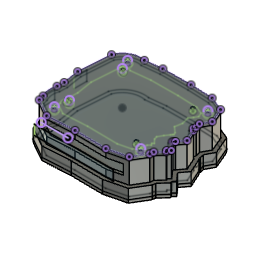
PCBPWM_v2 v1 (Autodesk Fusion 360 design; units mm, degrees)
Autodesk Fusion 360 part; units mm, degrees
sketch "pwm_pcb_larger-NPTH-drl_map" plane through (-62.4412, 140.8247, 0) normal (0, 0, 1) x (1, 0, 0)
  line L0 (167.8, -97.8) -> (171.4, -101.8)
  line L1 (171.4, -104.8) -> (169.4, -107)
  line L2 (85.4, -80) -> (87.4, -51.8)
  line L3 (122.4, -120.6) -> (98.6, -122)
  line L4 (94.9432, -49.9251) -> (114, -47.8)
  line L5 (88, -96.2) -> (85.4, -80)
  line L6 (168.6, -59) -> (166.2, -62.4)
  line L7 (173, -84.8) -> (172.2, -86)
  line L8 (141.4, -47.6) -> (161.2, -48.4)
  line L9 (172.2, -86) -> (169.4, -90)
  line L10 (169.4, -107) -> (168.8, -112)
  line L11 (170.4, -55.6) -> (168.6, -59)
  line L12 (168.8, -112) -> (165.2, -118)
  line L13 (171.4, -101.8) -> (170.2, -103)
  line L14 (166.2, -62.4) -> (168.2, -69.8)
  line L15 (172.6, -81.8) -> (173.6, -84)
  line L16 (89.2, -108.4) -> (92.4, -111.6)
  arc A0 (94.9432, -49.9251) -> (87.4, -51.8) centre (92.2153, -55.0617) ccw
  line L17 (92.4, -108.4) -> (89.2, -111.6)
  line L18 (91.491, -53.264) -> (94.691, -56.464)
  line L19 (166.8, -94.8) -> (167.8, -97.8)
  line L20 (114, -47.8) -> (141.4, -47.6)
  line L21 (161.2, -48.4) -> (168.6, -51.4)
  arc A1 (87.5716, -106.689) -> (88.2, -114.2) centre (93.4337, -109.9803) ccw
  line L22 (164.8, -110.2) -> (161.6, -113.4)
  line L23 (161.6, -110.2) -> (164.8, -113.4)
  line L24 (153, -121) -> (122.4, -120.6)
  line L25 (161.2, -52.2) -> (164.4, -55.4)
  line L26 (170.2, -103) -> (171.4, -104.8)
  line L27 (168.2, -69.8) -> (167, -76.8)
  line L28 (165.2, -118) -> (153, -121)
  line L29 (164.4, -52.2) -> (161.2, -55.4)
  line L30 (98.6, -122) -> (88.8, -116.4)
  line L31 (168.6, -51.4) -> (170.4, -55.6)
  line L32 (89.2, -108.4) -> (92.4, -111.6)
  line L33 (173.6, -84) -> (173, -84.8)
  line L34 (94.691, -53.264) -> (91.491, -56.464)
  line L35 (92.4, -108.4) -> (89.2, -111.6)
  line L36 (169.4, -90) -> (166.8, -94.8)
  line L37 (87.5716, -106.689) -> (88, -96.2)
  line L38 (167, -76.8) -> (172.6, -81.8)
  line L39 (88.8, -116.4) -> (88.2, -114.2)
  circle A2 centre (90.8, -110) radius 1.6
  circle A3 centre (163.2, -111.8) radius 1.6
  circle A4 centre (162.8, -53.8) radius 1.6
  circle A5 centre (93.091, -54.864) radius 1.6
  line L40 (176.1705, -43.6786) -> (181.4744, -56.0543)
  line L41 (181.4744, -56.0543) -> (177.1386, -64.2442)
  line L42 (177.1386, -64.2442) -> (177.0798, -64.3276)
  line L43 (177.0798, -64.3276) -> (178.4285, -69.318)
  line L44 (178.4285, -69.318) -> (177.7922, -73.0299)
  line L45 (177.7922, -73.0299) -> (180.8318, -75.7439)
  line L46 (180.8318, -75.7439) -> (185.1564, -85.2581)
  line L47 (185.1564, -85.2581) -> (181.1665, -90.5779)
  line L48 (181.1665, -90.5779) -> (180.4575, -91.6415)
  line L49 (180.4575, -91.6415) -> (178.3809, -94.6081)
  line L50 (178.3809, -94.6081) -> (185.1798, -102.1624)
  line L51 (185.1798, -102.1624) -> (183.068, -104.2742)
  line L52 (183.068, -104.2742) -> (184.0515, -105.7495)
  line L53 (184.0515, -105.7495) -> (178.9482, -111.3631)
  line L54 (178.9482, -111.3631) -> (178.4742, -115.3128)
  line L55 (178.4742, -115.3128) -> (171.6322, -126.7162)
  line L56 (171.6322, -126.7162) -> (154.147, -131.0158)
  line L57 (154.147, -131.0158) -> (122.6286, -130.6038)
  line L58 (122.6286, -130.6038) -> (96.2196, -132.1573)
  line L59 (96.2196, -132.1573) -> (80.2422, -123.0274)
  line L60 (80.2422, -123.0274) -> (78.976, -118.3845)
  arc A6 (77.6551, -104.4404) -> (78.976, -118.3845) centre (93.4337, -109.9803) ccw
  line L61 (77.6551, -104.4404) -> (77.9674, -96.7942)
  line L62 (77.9674, -96.7942) -> (75.3434, -80.4445)
  line L63 (75.3434, -80.4445) -> (77.5665, -49.0987)
  arc A7 (96.1108, -39.7329) -> (77.5665, -49.0987) centre (92.2153, -55.0617) ccw
  line L64 (96.1108, -39.7329) -> (113.4078, -37.8041)
  line L65 (113.4078, -37.8041) -> (141.5655, -37.5985)
  line L66 (141.5655, -37.5985) -> (163.3435, -38.4784)
  line L67 (163.3435, -38.4784) -> (176.1705, -43.6786)
  line L68 (180.2893, -64.7046) -> (181.4971, -69.1733)
  line L69 (181.4971, -69.1733) -> (181.0298, -71.8989)
  line L70 (181.0298, -71.8989) -> (183.3013, -73.927)
  line L71 (183.3013, -73.927) -> (188.6234, -85.6355)
  line L72 (188.6234, -85.6355) -> (183.6165, -92.3113)
  line L73 (183.6165, -92.3113) -> (182.9347, -93.334)
  line L74 (182.9347, -93.334) -> (182.2065, -94.3743)
  line L75 (182.2065, -94.3743) -> (189.3137, -102.2711)
  line L76 (189.3137, -102.2711) -> (186.9283, -104.6564)
  line L77 (186.9283, -104.6564) -> (187.8469, -106.0343)
  line L78 (187.8469, -106.0343) -> (181.8126, -112.672)
  line L79 (181.8126, -112.672) -> (181.3765, -116.3067)
  line L80 (181.3765, -116.3067) -> (173.5618, -129.3311)
  line L81 (173.5618, -129.3311) -> (154.4911, -134.0206)
  line L82 (154.4911, -134.0206) -> (122.6971, -133.605)
  line L83 (122.6971, -133.605) -> (95.5055, -135.2045)
  line L84 (95.5055, -135.2045) -> (77.6749, -125.0156)
  line L85 (77.6749, -125.0156) -> (76.1807, -119.5368)
  arc A8 (74.6751, -103.8887) -> (76.1807, -119.5368) centre (93.4337, -109.9803) ccw
  line L86 (74.6751, -103.8887) -> (74.9576, -96.9725)
  line L87 (74.9576, -96.9725) -> (72.3264, -80.5778)
  line L88 (72.3264, -80.5778) -> (74.6063, -48.4312)
  arc A9 (96.2964, -36.6936) -> (74.6063, -48.4312) centre (92.2153, -55.0617) ccw
  line L89 (96.2964, -36.6936) -> (113.2301, -34.8053)
  line L90 (113.2301, -34.8053) -> (141.6151, -34.5981)
  line L91 (141.6151, -34.5981) -> (163.9865, -35.502)
  line L92 (163.9865, -35.502) -> (178.4417, -41.3622)
  line L93 (178.4417, -41.3622) -> (184.7967, -56.1906)
  line L94 (184.7967, -56.1906) -> (180.2893, -64.7046)
  circle A10 centre (172.2599, -116.3067) radius 4.1 construction
  circle A11 centre (91.3496, -123.3578) radius 4.1 construction
  circle A12 centre (87.8304, -45.2941) radius 4.1 construction
  circle A13 centre (173.0302, -48.7764) radius 4.1 construction
  circle A14 centre (172.2599, -116.3067) radius 2
  circle A15 centre (173.0302, -48.7764) radius 2
  circle A16 centre (87.8304, -45.2941) radius 2
  circle A17 centre (91.3496, -123.3578) radius 2
  dimension "d1" = 3.2
  dimension "d2" = 3.2
  dimension "d3" = 3.2
  dimension "d4" = 3.2
  dimension "d5" = -10
  dimension "d6" = -13
  dimension "d11" = 8.2
  dimension "d12" = 8.2
  dimension "d13" = 8.2
  dimension "d14" = 8.2
  dimension "d15" = 4
  dimension "d16" = 4
  dimension "d17" = 4
  dimension "d18" = 4
  constraint midpoint L16 A2.centre
  constraint midpoint L23 A3.centre
  constraint midpoint L25 A4.centre
  constraint midpoint L18 A5.centre
  constraint concentric A10 A14
  constraint concentric A13 A15
  constraint concentric A12 A16
  constraint concentric A11 A17
  measures "d1" diameter of A2
  measures "d2" diameter of A3
  measures "d3" diameter of A5
  measures "d4" diameter of A4
  measures "d11" diameter of A10
  measures "d12" diameter of A11
  measures "d13" diameter of A12
  measures "d14" diameter of A13
  measures "d15" diameter of A14
  measures "d16" diameter of A15
  measures "d17" diameter of A16
  measures "d18" diameter of A17
extrude "Extrude1" add sketch "pwm_pcb_larger-NPTH-drl_map" against normal blind 31.75 contours L68 L69 L70 L71 L72 L73 L74 L75 L76 L77 L78 L79 L80 L81 L82 L83 L84 L85 A8 L86 L87 L88 A9 L89 L90 L91 L92 L93 L94 makes body 1
extrude "Extrude2" add sketch "pwm_pcb_larger-NPTH-drl_map" along normal blind 3 contours L0 L1 L2 L3 L4 L5 L6 L7 L8 L9 L10 L11 L12 L13 L14 L15 A0 L19 L20 L21 A1 L24 L26 L27 L28 L30 L31 L33 L36 L37 L38 L39 | L40 L41 L42 L43 L44 L45 L46 L47 L48 L49 L50 L51 L52 L53 L54 L55 L56 L57 L58 L59 L60 A6 L61 L62 L63 A7 L64 L65 L66 L67 | L68 L69 L70 L71 L72 L73 L74 L75 L76 L77 L78 L79 L80 L81 L82 L83 L84 L85 A8 L86 L87 L88 A9 L89 L90 L91 L92 L93 L94 bodies 1
sketch "Sketch2" plane through (0, 0, 3) normal (0, 0, 1) x (1, 0, 0)
  circle A0 centre (28.3588, 30.8247) radius 1.6
  circle A1 centre (100.7588, 29.0247) radius 1.6
  circle A2 centre (100.3588, 87.0247) radius 1.6
  circle A3 centre (30.6498, 85.9607) radius 1.6
  circle A4 centre (25.3892, 95.5306) radius 2
  circle A5 centre (110.589, 92.0483) radius 2
  circle A6 centre (28.9085, 17.467) radius 2
  circle A7 centre (109.8187, 24.518) radius 2
  arc A8 (33.8553, 104.1311) -> (12.1651, 92.3936) centre (29.7742, 85.763) ccw
  line L0 (12.1651, 92.3936) -> (9.8852, 60.2469)
  line L1 (9.8852, 60.2469) -> (12.5165, 43.8523)
  line L2 (12.5165, 43.8523) -> (12.234, 36.936)
  arc A9 (12.234, 36.936) -> (13.7395, 21.2879) centre (30.9925, 30.8444) ccw
  line L3 (13.7395, 21.2879) -> (15.2337, 15.8092)
  line L4 (15.2337, 15.8092) -> (33.0644, 5.6202)
  line L5 (33.0644, 5.6202) -> (60.256, 7.2197)
  line L6 (60.256, 7.2197) -> (92.05, 6.8041)
  line L7 (92.05, 6.8041) -> (111.1207, 11.4936)
  line L8 (111.1207, 11.4936) -> (118.9353, 24.518)
  line L9 (118.9353, 24.518) -> (119.3715, 28.1527)
  line L10 (119.3715, 28.1527) -> (125.4058, 34.7904)
  line L11 (125.4058, 34.7904) -> (124.4872, 36.1683)
  line L12 (124.4872, 36.1683) -> (126.8725, 38.5536)
  line L13 (126.8725, 38.5536) -> (119.7654, 46.4505)
  line L14 (119.7654, 46.4505) -> (120.4936, 47.4907)
  line L15 (120.4936, 47.4907) -> (121.1753, 48.5134)
  line L16 (121.1753, 48.5134) -> (126.1822, 55.1892)
  line L17 (126.1822, 55.1892) -> (120.8602, 66.8977)
  line L18 (120.8602, 66.8977) -> (118.5887, 68.9258)
  line L19 (118.5887, 68.9258) -> (119.0559, 71.6514)
  line L20 (119.0559, 71.6514) -> (117.8482, 76.1201)
  line L21 (117.8482, 76.1201) -> (122.3556, 84.6341)
  line L22 (122.3556, 84.6341) -> (116.0005, 99.4625)
  line L23 (116.0005, 99.4625) -> (101.5453, 105.3227)
  line L24 (101.5453, 105.3227) -> (79.1739, 106.2266)
  line L25 (79.1739, 106.2266) -> (50.789, 106.0195)
  line L26 (50.789, 106.0195) -> (33.8553, 104.1311)
sketch "Sketch3" plane through (0, 0, 0) normal (0, 1, 0) x (1, 0, 0)
  line L0 (26.2781, 5) -> (106.2781, 5)
  line L1 (106.2781, 5) -> (106.2781, 15)
  line L2 (106.2781, 15) -> (26.2781, 15)
  line L3 (26.2781, 15) -> (26.2781, 5)
  line L4 (60.256, 0) -> (33.0644, 0)
  dimension "d19" = 10
  dimension "d21" = 80
  dimension "d38" = 5
  constraint horizontal L0
  constraint vertical L1
  constraint horizontal L2
  constraint vertical L3
  measures "d19" distance of L0.start L2.end
  measures "d21" distance of L1 L3
  measures "d38" distance of origin L0
extrude "Extrude3" cut sketch "Sketch3" along normal blind 20 bodies 1
sketch "Sketch4" plane through (0, 0, 0) normal (1, 0, 0) x (0, 1, 0)
  line L0 (46.7893, -10) -> (33.7893, -10)
  line L1 (33.7893, -10) -> (33.7893, -20)
  line L2 (33.7893, -20) -> (46.7893, -20)
  line L3 (46.7893, -20) -> (46.7893, -10)
  line L4 (79.3949, -10) -> (66.3949, -10)
  line L5 (66.3949, -10) -> (66.3949, -20)
  line L6 (66.3949, -20) -> (79.3949, -20)
  line L7 (79.3949, -20) -> (79.3949, -10)
  dimension "d24" = 13
  dimension "d25" = 10
  dimension "d27" = 10
  dimension "d28" = 13
  dimension "d39" = 10
  dimension "d40" = 10
  constraint horizontal L0
  constraint vertical L1
  constraint horizontal L2
  constraint vertical L3
  constraint horizontal L4
  constraint vertical L5
  constraint horizontal L6
  constraint vertical L7
  measures "d24" distance of L0.start L0.end
  measures "d25" distance of L0.start L2.end
  measures "d27" distance of L4.start L6.end
  measures "d28" distance of L5 L7
  measures "d39" distance of origin L0
  measures "d40" distance of origin L4
extrude "Extrude4" cut sketch "Sketch4" along normal blind 30 bodies 1
sketch "Sketch6" plane through (0, 0, -31.75) normal (0, 0, -1) x (1, 0, 0)
  arc A0 (15.1253, -91.726) -> (33.6696, -101.0918) centre (29.7742, -85.763) ccw
  line L0 (15.1253, -91.726) -> (12.9022, -60.3803)
  line L1 (12.9022, -60.3803) -> (15.5262, -44.0305)
  line L2 (15.5262, -44.0305) -> (15.2139, -36.3843)
  arc A1 (16.5348, -22.4403) -> (15.2139, -36.3843) centre (30.9925, -30.8444) ccw
  line L3 (16.5348, -22.4403) -> (17.8011, -17.7974)
  line L4 (17.8011, -17.7974) -> (33.7785, -8.6674)
  line L5 (33.7785, -8.6674) -> (60.1874, -10.2209)
  line L6 (60.1874, -10.2209) -> (91.7059, -9.8089)
  line L7 (91.7059, -9.8089) -> (109.191, -14.1085)
  line L8 (109.191, -14.1085) -> (116.0331, -25.5119)
  line L9 (116.0331, -25.5119) -> (116.507, -29.4616)
  line L10 (116.507, -29.4616) -> (121.6103, -35.0753)
  line L11 (121.6103, -35.0753) -> (120.6268, -36.5505)
  line L12 (120.6268, -36.5505) -> (122.7386, -38.6623)
  line L13 (122.7386, -38.6623) -> (115.9397, -46.2166)
  line L14 (115.9397, -46.2166) -> (118.0163, -49.1832)
  line L15 (118.0163, -49.1832) -> (118.7254, -50.2468)
  line L16 (118.7254, -50.2468) -> (122.7153, -55.5666)
  line L17 (122.7153, -55.5666) -> (118.3907, -65.0808)
  line L18 (118.3907, -65.0808) -> (115.351, -67.7948)
  line L19 (115.351, -67.7948) -> (115.9874, -71.5068)
  line L20 (115.9874, -71.5068) -> (114.6386, -76.4972)
  line L21 (114.6386, -76.4972) -> (114.6974, -76.5805)
  line L22 (114.6974, -76.5805) -> (119.0332, -84.7704)
  line L23 (119.0332, -84.7704) -> (113.7294, -97.1461)
  line L24 (113.7294, -97.1461) -> (100.9023, -102.3463)
  line L25 (100.9023, -102.3463) -> (79.1243, -103.2262)
  line L26 (79.1243, -103.2262) -> (50.9666, -103.0207)
  line L27 (50.9666, -103.0207) -> (33.6696, -101.0918)
  arc A2 (12.1651, -92.3936) -> (33.8553, -104.1311) centre (29.7742, -85.763) ccw
  line L28 (33.8553, -104.1311) -> (50.789, -106.0195)
  line L29 (50.789, -106.0195) -> (79.1739, -106.2266)
  line L30 (79.1739, -106.2266) -> (101.5453, -105.3227)
  line L31 (101.5453, -105.3227) -> (116.0005, -99.4625)
  line L32 (116.0005, -99.4625) -> (122.3556, -84.6341)
  line L33 (122.3556, -84.6341) -> (117.8482, -76.1201)
  line L34 (117.8482, -76.1201) -> (119.0559, -71.6514)
  line L35 (119.0559, -71.6514) -> (118.5887, -68.9258)
  line L36 (118.5887, -68.9258) -> (120.8602, -66.8977)
  line L37 (120.8602, -66.8977) -> (126.1822, -55.1892)
  line L38 (126.1822, -55.1892) -> (121.1753, -48.5134)
  line L39 (121.1753, -48.5134) -> (120.4936, -47.4907)
  line L40 (120.4936, -47.4907) -> (119.7654, -46.4505)
  line L41 (119.7654, -46.4505) -> (126.8725, -38.5536)
  line L42 (126.8725, -38.5536) -> (124.4872, -36.1683)
  line L43 (124.4872, -36.1683) -> (125.4058, -34.7904)
  line L44 (125.4058, -34.7904) -> (119.3715, -28.1527)
  line L45 (119.3715, -28.1527) -> (118.9353, -24.518)
  line L46 (118.9353, -24.518) -> (111.1207, -11.4936)
  line L47 (111.1207, -11.4936) -> (92.05, -6.8041)
  line L48 (92.05, -6.8041) -> (60.256, -7.2197)
  line L49 (60.256, -7.2197) -> (33.0644, -5.6202)
  line L50 (33.0644, -5.6202) -> (15.2337, -15.8092)
  line L51 (15.2337, -15.8092) -> (13.7395, -21.2879)
  arc A3 (13.7395, -21.2879) -> (12.234, -36.936) centre (30.9925, -30.8444) ccw
  line L52 (12.234, -36.936) -> (12.5165, -43.8523)
  line L53 (12.5165, -43.8523) -> (9.8852, -60.2469)
  line L54 (9.8852, -60.2469) -> (12.1651, -92.3936)
  line L55 (8.5034, -43.6146) -> (5.8626, -60.0691)
  line L56 (5.8626, -60.0691) -> (8.2143, -93.2293)
  arc A4 (8.2143, -93.2293) -> (34.0407, -108.1766) centre (29.7742, -85.763) ccw
  line L57 (34.0407, -108.1766) -> (50.5521, -110.0178)
  line L58 (50.5521, -110.0178) -> (79.2401, -110.2272)
  line L59 (79.2401, -110.2272) -> (102.4027, -109.2914)
  line L60 (102.4027, -109.2914) -> (119.0287, -102.5511)
  line L61 (119.0287, -102.5511) -> (126.7853, -84.4523)
  line L62 (126.7853, -84.4523) -> (122.1209, -75.6418)
  line L63 (122.1209, -75.6418) -> (123.1473, -71.8442)
  line L64 (123.1473, -71.8442) -> (122.9055, -70.4339)
  line L65 (122.9055, -70.4339) -> (124.1529, -69.3201)
  line L66 (124.1529, -69.3201) -> (130.8048, -54.686)
  line L67 (130.8048, -54.686) -> (124.8639, -46.7648)
  line L68 (124.8639, -46.7648) -> (132.3844, -38.4087)
  line L69 (132.3844, -38.4087) -> (129.6344, -35.6586)
  line L70 (129.6344, -35.6586) -> (130.4664, -34.4107)
  line L71 (130.4664, -34.4107) -> (123.1907, -26.4075)
  line L72 (123.1907, -26.4075) -> (122.805, -23.1929)
  line L73 (122.805, -23.1929) -> (113.6935, -8.0072)
  line L74 (113.6935, -8.0072) -> (92.5088, -2.7978)
  line L75 (92.5088, -2.7978) -> (60.3474, -3.2182)
  line L76 (60.3474, -3.2182) -> (32.1122, -1.5573)
  line L77 (32.1122, -1.5573) -> (11.8106, -13.1582)
  line L78 (11.8106, -13.1582) -> (10.0012, -19.7927)
  arc A5 (10.0012, -19.7927) -> (8.2587, -37.6228) centre (30.9925, -30.8444) ccw
  line L79 (8.2587, -37.6228) -> (8.5034, -43.6146)
  arc A6 (11.869, -92.4582) -> (33.8714, -104.4348) centre (29.7742, -85.763) ccw
  line L80 (33.8714, -104.4348) -> (50.7712, -106.3193)
  line L81 (50.7712, -106.3193) -> (79.1789, -106.5267)
  line L82 (79.1789, -106.5267) -> (101.6096, -105.6204)
  line L83 (101.6096, -105.6204) -> (116.2276, -99.6942)
  line L84 (116.2276, -99.6942) -> (122.6878, -84.6204)
  line L85 (122.6878, -84.6204) -> (118.1686, -76.0842)
  line L86 (118.1686, -76.0842) -> (119.3628, -71.6658)
  line L87 (119.3628, -71.6658) -> (118.9124, -69.0389)
  line L88 (118.9124, -69.0389) -> (121.1072, -67.0794)
  line L89 (121.1072, -67.0794) -> (126.5289, -55.1515)
  line L90 (126.5289, -55.1515) -> (121.4203, -48.3401)
  line L91 (121.4203, -48.3401) -> (120.7413, -47.3215)
  line L92 (120.7413, -47.3215) -> (120.148, -46.4738)
  line L93 (120.148, -46.4738) -> (127.2859, -38.5428)
  line L94 (127.2859, -38.5428) -> (124.8732, -36.1301)
  line L95 (124.8732, -36.1301) -> (125.7853, -34.762)
  line L96 (125.7853, -34.762) -> (119.6579, -28.0218)
  line L97 (119.6579, -28.0218) -> (119.2255, -24.4187)
  line L98 (119.2255, -24.4187) -> (111.3136, -11.2322)
  line L99 (111.3136, -11.2322) -> (92.0844, -6.5036)
  line L100 (92.0844, -6.5036) -> (60.2628, -6.9196)
  line L101 (60.2628, -6.9196) -> (32.993, -5.3155)
  line L102 (32.993, -5.3155) -> (14.977, -15.6103)
  line L103 (14.977, -15.6103) -> (13.4596, -21.1743)
  arc A7 (13.4596, -21.1743) -> (11.9359, -36.9893) centre (30.9925, -30.8444) ccw
  line L104 (11.9359, -36.9893) -> (12.2155, -43.8344)
  line L105 (12.2155, -43.8344) -> (9.5835, -60.2336)
  line L106 (9.5835, -60.2336) -> (11.869, -92.4582)
  dimension "d41" = 4
  dimension "d42" = 0.3
extrude "Extrude7" add sketch "Sketch6" along normal blind 3 separate body contours A0 L0 L1 L2 A1 L3 L4 L5 L6 L7 L8 L9 L10 L11 L12 L13 L14 L15 L16 L17 L18 L19 L20 L21 L22 L23 L24 L25 L26 L27 | A2 L28 L29 L30 L31 L32 L33 L34 L35 L36 L37 L38 L39 L40 L41 L42 L43 L44 L45 L46 L47 L48 L49 L50 L51 A3 L52 L53 L54 | L55 L56 A4 L57 L58 L59 L60 L61 L62 L63 L64 L65 L66 L67 L68 L69 L70 L71 L72 L73 L74 L75 L76 L77 L78 A5 L79 | A6 L80 L81 L82 L83 L84 L85 L86 L87 L88 L89 L90 L91 L92 L93 L94 L95 L96 L97 L98 L99 L100 L101 L102 L103 A7 L104 L105 L106 makes body 2
extrude "Extrude8" add sketch "Sketch6" against normal blind 10 contours L55 L56 A4 L57 L58 L59 L60 L61 L62 L63 L64 L65 L66 L67 L68 L69 L70 L71 L72 L73 L74 L75 L76 L77 L78 A5 L79 bodies 2
move_body "Move1" bodies 2 to x (1, 0, 0) y (0, 1, 0) z (0, 0, 1) at (0, 0, -60)
move_body "Move2" bodies 2 to x (1, 0, 0) y (0, 1, 0) z (0, 0, 1) at (0, 0, 60)
named bodies: "Lower", "upper"
